Autodesk Fusion 360 part; units mm, degrees
note: some values were not read from the file. Set by a fixed rule: which sketch regions a step uses.
(part 15 of 59)
  spline S83 degree 5 poles (-2.755, -18.3773) (-2.7539, -18.3749) (-2.7515, -18.37) (-2.748, -18.3627) (-2.7434, -18.353) (-2.7376, -18.3408) (-2.7319, -18.3287) (-2.7262, -18.3165) (-2.7205, -18.3044) (-2.7149, -18.2924) (-2.7092, -18.2803) (-2.7036, -18.2683) (-2.6981, -18.2563) (-2.6925, -18.2443) (-2.687, -18.2323) (-2.6815, -18.2204) (-2.6761, -18.2085) (-2.6707, -18.1966) (-2.6653, -18.1847) (-2.6599, -18.1728) (-2.6545, -18.161) (-2.6492, -18.1492) (-2.6439, -18.1374) (-2.6387, -18.1256) (-2.6335, -18.1139) (-2.6283, -18.1022) (-2.6231, -18.0905) (-2.6179, -18.0788) (-2.6128, -18.0672) (-2.6077, -18.0555) (-2.6027, -18.0439) (-2.5977, -18.0324) (-2.5927, -18.0208) (-2.5877, -18.0093) (-2.5827, -17.9978) (-2.5778, -17.9863) (-2.5729, -17.9749) (-2.5681, -17.9634) (-2.5632, -17.952) (-2.5584, -17.9407) (-2.5537, -17.9293) (-2.5489, -17.918) (-2.5442, -17.9067) (-2.5395, -17.8954) (-2.5348, -17.8841) (-2.5302, -17.8729) (-2.5256, -17.8617) (-2.521, -17.8506) (-2.5165, -17.8394) (-2.5119, -17.8283) (-2.5074, -17.8172) (-2.503, -17.8061) (-2.4985, -17.7951) (-2.4941, -17.7841) (-2.4897, -17.7731) (-2.4854, -17.7621) (-2.481, -17.7512) (-2.4767, -17.7403) (-2.4725, -17.7294) (-2.4682, -17.7186) (-2.464, -17.7078) (-2.4598, -17.697) (-2.4557, -17.6862) (-2.4515, -17.6755) (-2.4474, -17.6648) (-2.4433, -17.6541) (-2.4393, -17.6435) (-2.4353, -17.6329) (-2.4313, -17.6223) (-2.4273, -17.6118) (-2.4234, -17.6012) (-2.4194, -17.5907) (-2.4156, -17.5803) (-2.4117, -17.5699) (-2.4079, -17.5595) (-2.4041, -17.5491) (-2.4003, -17.5388) (-2.3965, -17.5284) (-2.3928, -17.5182) (-2.3891, -17.5079) (-2.3855, -17.4977) (-2.3818, -17.4875) (-2.3782, -17.4774) (-2.3746, -17.4673) (-2.3711, -17.4572) (-2.3675, -17.4471) (-2.364, -17.4371) (-2.3606, -17.4271) (-2.3571, -17.4172) (-2.3537, -17.4073) (-2.3503, -17.3974) (-2.3469, -17.3875) (-2.3436, -17.3777) (-2.3403, -17.368) (-2.337, -17.3582) (-2.3337, -17.3485) (-2.3305, -17.3388) (-2.3273, -17.3292) (-2.3241, -17.3196) (-2.321, -17.31) (-2.3178, -17.3005) (-2.3147, -17.291) (-2.3117, -17.2815) (-2.3086, -17.2721) (-2.3056, -17.2627) (-2.3026, -17.2534) (-2.2996, -17.2441) (-2.2967, -17.2348) (-2.2938, -17.2255) (-2.2909, -17.2163) (-2.288, -17.2072) (-2.2852, -17.1981) (-2.2824, -17.189) (-2.2796, -17.1799) (-2.2769, -17.1709) (-2.2741, -17.1619) (-2.2714, -17.153) (-2.2688, -17.1441) (-2.2661, -17.1353) (-2.2635, -17.1265) (-2.2609, -17.1177) (-2.2583, -17.109) (-2.2558, -17.1003) (-2.2533, -17.0917) (-2.2508, -17.083) (-2.2483, -17.0745) (-2.2458, -17.066) (-2.2434, -17.0575) (-2.241, -17.0491) (-2.2387, -17.0407) (-2.2363, -17.0323) (-2.234, -17.024) (-2.2317, -17.0158) (-2.2295, -17.0075) (-2.2272, -16.9994) (-2.225, -16.9912) (-2.2228, -16.9832) (-2.2207, -16.9751) (-2.2185, -16.9671) (-2.2164, -16.9592) (-2.2143, -16.9513) (-2.2123, -16.9434) (-2.2102, -16.9356) (-2.2082, -16.9279) (-2.2062, -16.9202) (-2.2043, -16.9125) (-2.2023, -16.9049) (-2.2004, -16.8973) (-2.1985, -16.8898) (-2.1967, -16.8823) (-2.1948, -16.8749) (-2.193, -16.8675) (-2.1912, -16.8602) (-2.1895, -16.8529) (-2.1877, -16.8457) (-2.186, -16.8386) (-2.1843, -16.8314) (-2.1827, -16.8244) (-2.181, -16.8174) (-2.1794, -16.8104) (-2.1778, -16.8035) (-2.1762, -16.7967) (-2.1747, -16.7899) (-2.1731, -16.7831) (-2.1716, -16.7764) (-2.1702, -16.7698) (-2.1687, -16.7632) (-2.1673, -16.7567) (-2.1659, -16.7502) (-2.1645, -16.7438) (-2.1631, -16.7374) (-2.1618, -16.7311) (-2.1605, -16.7249) (-2.1592, -16.7187) (-2.1579, -16.7126) (-2.1567, -16.7065) (-2.1554, -16.7005) (-2.1542, -16.6946) (-2.153, -16.6887) (-2.1519, -16.6829) (-2.1507, -16.6771) (-2.1496, -16.6714) (-2.1485, -16.6658) (-2.1475, -16.6602) (-2.1464, -16.6547) (-2.1454, -16.6493) (-2.1444, -16.6439) (-2.1434, -16.6386) (-2.1424, -16.6334) (-2.1415, -16.6282) (-2.1406, -16.6231) (-2.1397, -16.618) (-2.1388, -16.6131) (-2.138, -16.6081) (-2.1371, -16.6033) (-2.1363, -16.5985) (-2.1355, -16.5938) (-2.1347, -16.5892) (-2.134, -16.5847) (-2.1332, -16.5802) (-2.1325, -16.5758) (-2.1318, -16.5714) (-2.1312, -16.5672) (-2.1305, -16.563) (-2.1299, -16.5589) (-2.1292, -16.5549) (-2.1286, -16.5509) (-2.1281, -16.547) (-2.1275, -16.5432) (-2.127, -16.5395) (-2.1264, -16.5359) (-2.1259, -16.5323) (-2.1254, -16.5289) (-2.125, -16.5255) (-2.1245, -16.5222) (-2.1241, -16.5189) (-2.1237, -16.5158) (-2.1233, -16.5128) (-2.1229, -16.5098) (-2.1225, -16.5069) (-2.1222, -16.5041) (-2.1219, -16.5015) (-2.1215, -16.4989) (-2.1212, -16.4963) (-2.121, -16.4939) (-2.1207, -16.4916) (-2.1204, -16.4894) (-2.1202, -16.4873) (-2.12, -16.4852) (-2.1198, -16.4833) (-2.1196, -16.4815) (-2.1194, -16.4798) (-2.1192, -16.4781) (-2.1191, -16.4766) (-2.1189, -16.4752) (-2.1188, -16.4739) (-2.1187, -16.4727) (-2.1186, -16.4716) (-2.1185, -16.4706) (-2.1184, -16.4698) (-2.1184, -16.469) (-2.1183, -16.4685) (-2.1183, -16.4682) (-2.1183, -16.468) (-2.1183, -16.4679) knots -1 -1 -1 -1 -1 -1 -0.99583333 -0.99166667 -0.9875 -0.98333333 -0.97916667 -0.975 -0.97083333 -0.96666667 -0.9625 -0.95833333 -0.95416667 -0.95 -0.94583333 -0.94166667 -0.9375 -0.93333333 -0.92916667 -0.925 -0.92083333 -0.91666667 -0.9125 -0.90833333 -0.90416667 -0.9 -0.89583333 -0.89166667 -0.8875 -0.88333333 -0.87916667 -0.875 -0.87083333 -0.86666667 -0.8625 -0.85833333 -0.85416667 -0.85 -0.84583333 -0.84166667 -0.8375 -0.83333333 -0.82916667 -0.825 -0.82083333 -0.81666667 -0.8125 -0.80833333 -0.80416667 -0.8 -0.79583333 -0.79166667 -0.7875 -0.78333333 -0.77916667 -0.775 -0.77083333 -0.76666667 -0.7625 -0.75833333 -0.75416667 -0.75 -0.74583333 -0.74166667 -0.7375 -0.73333333 -0.72916667 -0.725 -0.72083333 -0.71666667 -0.7125 -0.70833333 -0.70416667 -0.7 -0.69583333 -0.69166667 -0.6875 -0.68333333 -0.67916667 -0.675 -0.67083333 -0.66666667 -0.6625 -0.65833333 -0.65416667 -0.65 -0.64583333 -0.64166667 -0.6375 -0.63333333 -0.62916667 -0.625 -0.62083333 -0.61666667 -0.6125 -0.60833333 -0.60416667 -0.6 -0.59583333 -0.59166667 -0.5875 -0.58333333 -0.57916667 -0.575 -0.57083333 -0.56666667 -0.5625 -0.55833333 -0.55416667 -0.55 -0.54583333 -0.54166667 -0.5375 -0.53333333 -0.52916667 -0.525 -0.52083333 -0.51666667 -0.5125 -0.50833333 -0.50416667 -0.5 -0.49583333 -0.49166667 -0.4875 -0.48333333 -0.47916667 -0.475 -0.47083333 -0.46666667 -0.4625 -0.45833333 -0.45416667 -0.45 -0.44583333 -0.44166667 -0.4375 -0.43333333 -0.42916667 -0.425 -0.42083333 -0.41666667 -0.4125 -0.40833333 -0.40416667 -0.4 -0.39583333 -0.39166667 -0.3875 -0.38333333 -0.37916667 -0.375 -0.37083333 -0.36666667 -0.3625 -0.35833333 -0.35416667 -0.35 -0.34583333 -0.34166667 -0.3375 -0.33333333 -0.32916667 -0.325 -0.32083333 -0.31666667 -0.3125 -0.30833333 -0.30416667 -0.3 -0.29583333 -0.29166667 -0.2875 -0.28333333 -0.27916667 -0.275 -0.27083333 -0.26666667 -0.2625 -0.25833333 -0.25416667 -0.25 -0.24583333 -0.24166667 -0.2375 -0.23333333 -0.22916667 -0.225 -0.22083333 -0.21666667 -0.2125 -0.20833333 -0.20416667 -0.2 -0.19583333 -0.19166667 -0.1875 -0.18333333 -0.17916667 -0.175 -0.17083333 -0.16666667 -0.1625 -0.15833333 -0.15416667 -0.15 -0.14583333 -0.14166667 -0.1375 -0.13333333 -0.12916667 -0.125 -0.12083333 -0.11666667 -0.1125 -0.10833333 -0.10416667 -0.1 -0.09583333 -0.09166667 -0.0875 -0.08333333 -0.07916667 -0.075 -0.07083333 -0.06666667 -0.0625 -0.05833333 -0.05416667 -0.05 -0.04583333 -0.04166667 -0.0375 -0.03333333 -0.02916667 -0.025 -0.02083333 -0.01666667 -0.0125 -0.00833333 -0.00416667 0 0 0 0 0 0
  spline S84 degree 5 poles (26.1461, -0.1495) (26.1462, -0.1495) (26.1464, -0.1496) (26.1467, -0.1497) (26.1471, -0.15) (26.1478, -0.1503) (26.1486, -0.1506) (26.1495, -0.151) (26.1504, -0.1515) (26.1515, -0.152) (26.1527, -0.1526) (26.154, -0.1531) (26.1554, -0.1538) (26.1569, -0.1544) (26.1585, -0.1551) (26.1602, -0.1559) (26.1619, -0.1567) (26.1638, -0.1575) (26.1658, -0.1583) (26.1678, -0.1592) (26.17, -0.1602) (26.1722, -0.1611) (26.1745, -0.1621) (26.1769, -0.1631) (26.1794, -0.1642) (26.182, -0.1653) (26.1847, -0.1664) (26.1874, -0.1676) (26.1903, -0.1687) (26.1932, -0.1699) (26.1962, -0.1712) (26.1993, -0.1724) (26.2024, -0.1737) (26.2057, -0.175) (26.209, -0.1764) (26.2124, -0.1778) (26.2159, -0.1791) (26.2195, -0.1806) (26.2231, -0.182) (26.2269, -0.1834) (26.2307, -0.1849) (26.2345, -0.1864) (26.2385, -0.188) (26.2425, -0.1895) (26.2466, -0.1911) (26.2508, -0.1927) (26.255, -0.1943) (26.2594, -0.1959) (26.2638, -0.1975) (26.2682, -0.1992) (26.2728, -0.2009) (26.2774, -0.2026) (26.282, -0.2043) (26.2868, -0.206) (26.2916, -0.2077) (26.2965, -0.2095) (26.3015, -0.2113) (26.3065, -0.2131) (26.3116, -0.2149) (26.3167, -0.2167) (26.322, -0.2185) (26.3273, -0.2204) (26.3326, -0.2222) (26.338, -0.2241) (26.3435, -0.226) (26.3491, -0.2279) (26.3547, -0.2298) (26.3604, -0.2317) (26.3661, -0.2336) (26.3719, -0.2356) (26.3778, -0.2375) (26.3837, -0.2395) (26.3897, -0.2414) (26.3958, -0.2434) (26.4019, -0.2454) (26.4081, -0.2474) (26.4144, -0.2494) (26.4207, -0.2514) (26.427, -0.2534) (26.4335, -0.2555) (26.4399, -0.2575) (26.4465, -0.2596) (26.4531, -0.2616) (26.4598, -0.2637) (26.4665, -0.2657) (26.4733, -0.2678) (26.4801, -0.2699) (26.487, -0.272) (26.4939, -0.274) (26.5009, -0.2761) (26.508, -0.2782) (26.5151, -0.2803) (26.5223, -0.2824) (26.5296, -0.2845) (26.5368, -0.2867) (26.5442, -0.2888) (26.5516, -0.2909) (26.559, -0.293) (26.5665, -0.2952) (26.5741, -0.2973) (26.5817, -0.2994) (26.5894, -0.3016) (26.5971, -0.3037) (26.6049, -0.3058) (26.6127, -0.308) (26.6206, -0.3101) (26.6286, -0.3123) (26.6365, -0.3144) (26.6446, -0.3166) (26.6527, -0.3187) (26.6608, -0.3208) (26.669, -0.323) (26.6773, -0.3251) (26.6856, -0.3273) (26.6939, -0.3294) (26.7023, -0.3316) (26.7108, -0.3337) (26.7193, -0.3359) (26.7278, -0.338) (26.7364, -0.3402) (26.7451, -0.3423) (26.7537, -0.3445) (26.7625, -0.3466) (26.7713, -0.3487) (26.7801, -0.3509) (26.789, -0.353) (26.798, -0.3551) (26.8069, -0.3573) (26.816, -0.3594) (26.8251, -0.3615) (26.8342, -0.3636) (26.8434, -0.3658) (26.8526, -0.3679) (26.8619, -0.37) (26.8712, -0.3721) (26.8806, -0.3742) (26.89, -0.3763) (26.8994, -0.3784) (26.9089, -0.3805) (26.9185, -0.3826) (26.9281, -0.3847) (26.9377, -0.3867) (26.9474, -0.3888) (26.9571, -0.3909) (26.9669, -0.3929) (26.9767, -0.395) (26.9866, -0.3971) (26.9965, -0.3991) (27.0064, -0.4011) (27.0164, -0.4032) (27.0265, -0.4052) (27.0365, -0.4072) (27.0467, -0.4093) (27.0568, -0.4113) (27.0671, -0.4133) (27.0773, -0.4153) (27.0876, -0.4173) (27.0979, -0.4193) (27.1083, -0.4213) (27.1188, -0.4232) (27.1292, -0.4252) (27.1397, -0.4272) (27.1503, -0.4291) (27.1609, -0.4311) (27.1715, -0.433) (27.1822, -0.4349) (27.1929, -0.4368) (27.2037, -0.4388) (27.2145, -0.4407) (27.2253, -0.4426) (27.2362, -0.4445) (27.2471, -0.4463) (27.2581, -0.4482) (27.2691, -0.4501) (27.2801, -0.4519) (27.2912, -0.4538) (27.3023, -0.4556) (27.3135, -0.4574) (27.3247, -0.4593) (27.3359, -0.4611) (27.3472, -0.4629) (27.3585, -0.4647) (27.3699, -0.4665) (27.3813, -0.4682) (27.3927, -0.47) (27.4042, -0.4718) (27.4157, -0.4735) (27.4273, -0.4752) (27.4388, -0.477) (27.4505, -0.4787) (27.4621, -0.4804) (27.4738, -0.4821) (27.4856, -0.4838) (27.4974, -0.4854) (27.5092, -0.4871) (27.521, -0.4887) (27.5329, -0.4904) (27.5449, -0.492) (27.5568, -0.4936) (27.5688, -0.4952) (27.5809, -0.4968) (27.5929, -0.4984) (27.605, -0.5) (27.6172, -0.5016) (27.6294, -0.5031) (27.6416, -0.5047) (27.6539, -0.5062) (27.6661, -0.5077) (27.6785, -0.5092) (27.6908, -0.5107) (27.7032, -0.5122) (27.7157, -0.5136) (27.7281, -0.5151) (27.7406, -0.5165) (27.7532, -0.518) (27.7658, -0.5194) (27.7784, -0.5208) (27.791, -0.5222) (27.8037, -0.5236) (27.8164, -0.5249) (27.8291, -0.5263) (27.8419, -0.5276) (27.8547, -0.529) (27.8676, -0.5303) (27.8805, -0.5316) (27.8934, -0.5329) (27.9063, -0.5342) (27.9193, -0.5354) (27.9323, -0.5367) (27.9454, -0.5379) (27.9585, -0.5391) (27.9716, -0.5404) (27.9848, -0.5415) (27.9979, -0.5427) (28.0112, -0.5439) (28.0244, -0.5451) (28.0377, -0.5462) (28.051, -0.5473) (28.0644, -0.5484) (28.0777, -0.5495) (28.0911, -0.5506) (28.1019, -0.5515) (28.11, -0.5521) (28.1154, -0.5525) (28.1181, -0.5527) knots 0 0 0 0 0 0 0.00416667 0.00833333 0.0125 0.01666667 0.02083333 0.025 0.02916667 0.03333333 0.0375 0.04166667 0.04583333 0.05 0.05416667 0.05833333 0.0625 0.06666667 0.07083333 0.075 0.07916667 0.08333333 0.0875 0.09166667 0.09583333 0.1 0.10416667 0.10833333 0.1125 0.11666667 0.12083333 0.125 0.12916667 0.13333333 0.1375 0.14166667 0.14583333 0.15 0.15416667 0.15833333 0.1625 0.16666667 0.17083333 0.175 0.17916667 0.18333333 0.1875 0.19166667 0.19583333 0.2 0.20416667 0.20833333 0.2125 0.21666667 0.22083333 0.225 0.22916667 0.23333333 0.2375 0.24166667 0.24583333 0.25 0.25416667 0.25833333 0.2625 0.26666667 0.27083333 0.275 0.27916667 0.28333333 0.2875 0.29166667 0.29583333 0.3 0.30416667 0.30833333 0.3125 0.31666667 0.32083333 0.325 0.32916667 0.33333333 0.3375 0.34166667 0.34583333 0.35 0.35416667 0.35833333 0.3625 0.36666667 0.37083333 0.375 0.37916667 0.38333333 0.3875 0.39166667 0.39583333 0.4 0.40416667 0.40833333 0.4125 0.41666667 0.42083333 0.425 0.42916667 0.43333333 0.4375 0.44166667 0.44583333 0.45 0.45416667 0.45833333 0.4625 0.46666667 0.47083333 0.475 0.47916667 0.48333333 0.4875 0.49166667 0.49583333 0.5 0.50416667 0.50833333 0.5125 0.51666667 0.52083333 0.525 0.52916667 0.53333333 0.5375 0.54166667 0.54583333 0.55 0.55416667 0.55833333 0.5625 0.56666667 0.57083333 0.575 0.57916667 0.58333333 0.5875 0.59166667 0.59583333 0.6 0.60416667 0.60833333 0.6125 0.61666667 0.62083333 0.625 0.62916667 0.63333333 0.6375 0.64166667 0.64583333 0.65 0.65416667 0.65833333 0.6625 0.66666667 0.67083333 0.675 0.67916667 0.68333333 0.6875 0.69166667 0.69583333 0.7 0.70416667 0.70833333 0.7125 0.71666667 0.72083333 0.725 0.72916667 0.73333333 0.7375 0.74166667 0.74583333 0.75 0.75416667 0.75833333 0.7625 0.76666667 0.77083333 0.775 0.77916667 0.78333333 0.7875 0.79166667 0.79583333 0.8 0.80416667 0.80833333 0.8125 0.81666667 0.82083333 0.825 0.82916667 0.83333333 0.8375 0.84166667 0.84583333 0.85 0.85416667 0.85833333 0.8625 0.86666667 0.87083333 0.875 0.87916667 0.88333333 0.8875 0.89166667 0.89583333 0.9 0.90416667 0.90833333 0.9125 0.91666667 0.92083333 0.925 0.92916667 0.93333333 0.9375 0.94166667 0.94583333 0.95 0.95416667 0.95833333 0.9625 0.96666667 0.97083333 0.975 0.97916667 0.98333333 0.9875 0.99166667 0.99583333 1 1 1 1 1 1
  arc A88 (18.6136, 37.2898) -> (17.8246, 37.863) centre (0, 12.5) ccw
  spline S85 degree 5 poles (5.9675, 42.9202) (5.9661, 42.9179) (5.9633, 42.9133) (5.959, 42.9064) (5.9534, 42.8972) (5.9464, 42.8857) (5.9394, 42.8742) (5.9325, 42.8628) (5.9255, 42.8513) (5.9187, 42.8399) (5.9118, 42.8285) (5.905, 42.8171) (5.8982, 42.8058) (5.8914, 42.7944) (5.8847, 42.7831) (5.878, 42.7718) (5.8713, 42.7605) (5.8647, 42.7492) (5.8581, 42.738) (5.8515, 42.7268) (5.8449, 42.7156) (5.8384, 42.7044) (5.8319, 42.6932) (5.8255, 42.6821) (5.8191, 42.6709) (5.8127, 42.6598) (5.8063, 42.6487) (5.8, 42.6377) (5.7937, 42.6266) (5.7874, 42.6156) (5.7811, 42.6046) (5.7749, 42.5936) (5.7688, 42.5826) (5.7626, 42.5717) (5.7565, 42.5608) (5.7504, 42.5499) (5.7443, 42.539) (5.7383, 42.5281) (5.7323, 42.5173) (5.7263, 42.5065) (5.7204, 42.4957) (5.7145, 42.4849) (5.7086, 42.4742) (5.7028, 42.4634) (5.697, 42.4527) (5.6912, 42.4421) (5.6854, 42.4314) (5.6797, 42.4208) (5.674, 42.4102) (5.6683, 42.3996) (5.6627, 42.389) (5.6571, 42.3785) (5.6515, 42.368) (5.646, 42.3575) (5.6405, 42.347) (5.635, 42.3366) (5.6296, 42.3262) (5.6242, 42.3158) (5.6188, 42.3054) (5.6134, 42.2951) (5.6081, 42.2847) (5.6028, 42.2745) (5.5975, 42.2642) (5.5923, 42.254) (5.5871, 42.2437) (5.5819, 42.2336) (5.5768, 42.2234) (5.5717, 42.2133) (5.5666, 42.2032) (5.5615, 42.1931) (5.5565, 42.183) (5.5515, 42.173) (5.5466, 42.163) (5.5416, 42.153) (5.5367, 42.1431) (5.5319, 42.1332) (5.527, 42.1233) (5.5222, 42.1134) (5.5175, 42.1036) (5.5127, 42.0938) (5.508, 42.084) (5.5033, 42.0743) (5.4987, 42.0646) (5.494, 42.0549) (5.4895, 42.0452) (5.4849, 42.0356) (5.4804, 42.026) (5.4759, 42.0165) (5.4714, 42.0069) (5.467, 41.9974) (5.4625, 41.9879) (5.4582, 41.9785) (5.4538, 41.9691) (5.4495, 41.9597) (5.4452, 41.9504) (5.441, 41.941) (5.4367, 41.9318) (5.4325, 41.9225) (5.4284, 41.9133) (5.4242, 41.9041) (5.4201, 41.895) (5.4161, 41.8858) (5.412, 41.8767) (5.408, 41.8677) (5.404, 41.8587) (5.4001, 41.8497) (5.3961, 41.8407) (5.3922, 41.8318) (5.3884, 41.8229) (5.3846, 41.8141) (5.3807, 41.8053) (5.377, 41.7965) (5.3732, 41.7878) (5.3695, 41.779) (5.3658, 41.7704) (5.3622, 41.7617) (5.3586, 41.7531) (5.355, 41.7446) (5.3514, 41.7361) (5.3479, 41.7276) (5.3444, 41.7191) (5.3409, 41.7107) (5.3375, 41.7023) (5.3341, 41.694) (5.3307, 41.6857) (5.3273, 41.6775) (5.324, 41.6692) (5.3207, 41.6611) (5.3175, 41.6529) (5.3143, 41.6448) (5.3111, 41.6368) (5.3079, 41.6288) (5.3047, 41.6208) (5.3016, 41.6129) (5.2986, 41.605) (5.2955, 41.5971) (5.2925, 41.5893) (5.2895, 41.5815) (5.2865, 41.5738) (5.2836, 41.5661) (5.2807, 41.5585) (5.2778, 41.5509) (5.275, 41.5433) (5.2722, 41.5358) (5.2694, 41.5284) (5.2666, 41.521) (5.2639, 41.5136) (5.2612, 41.5063) (5.2586, 41.499) (5.2559, 41.4918) (5.2533, 41.4846) (5.2508, 41.4774) (5.2482, 41.4703) (5.2457, 41.4633) (5.2432, 41.4563) (5.2408, 41.4493) (5.2383, 41.4424) (5.2359, 41.4356) (5.2336, 41.4288) (5.2312, 41.422) (5.2289, 41.4153) (5.2266, 41.4087) (5.2244, 41.4021) (5.2222, 41.3955) (5.22, 41.389) (5.2178, 41.3826) (5.2157, 41.3762) (5.2136, 41.3699) (5.2115, 41.3636) (5.2094, 41.3573) (5.2074, 41.3512) (5.2054, 41.3451) (5.2035, 41.339) (5.2015, 41.333) (5.1996, 41.327) (5.1978, 41.3211) (5.1959, 41.3153) (5.1941, 41.3095) (5.1923, 41.3038) (5.1905, 41.2981) (5.1888, 41.2925) (5.1871, 41.2869) (5.1854, 41.2815) (5.1838, 41.276) (5.1822, 41.2707) (5.1806, 41.2654) (5.179, 41.2601) (5.1775, 41.2549) (5.176, 41.2498) (5.1745, 41.2448) (5.173, 41.2398) (5.1716, 41.2349) (5.1702, 41.23) (5.1689, 41.2252) (5.1675, 41.2205) (5.1662, 41.2158) (5.1649, 41.2112) (5.1637, 41.2067) (5.1625, 41.2023) (5.1613, 41.1979) (5.1601, 41.1936) (5.1589, 41.1893) (5.1578, 41.1852) (5.1567, 41.1811) (5.1557, 41.1771) (5.1546, 41.1731) (5.1536, 41.1693) (5.1527, 41.1655) (5.1517, 41.1617) (5.1508, 41.1581) (5.1499, 41.1545) (5.149, 41.1511) (5.1481, 41.1477) (5.1473, 41.1443) (5.1465, 41.1411) (5.1458, 41.1379) (5.145, 41.1349) (5.1443, 41.1319) (5.1436, 41.129) (5.143, 41.1262) (5.1423, 41.1234) (5.1417, 41.1208) (5.1411, 41.1182) (5.1406, 41.1158) (5.14, 41.1134) (5.1395, 41.1111) (5.139, 41.1089) (5.1386, 41.1069) (5.1381, 41.1049) (5.1377, 41.103) (5.1374, 41.1012) (5.137, 41.0995) (5.1367, 41.0979) (5.1363, 41.0964) (5.1361, 41.095) (5.1358, 41.0937) (5.1356, 41.0925) (5.1354, 41.0915) (5.1352, 41.0905) (5.135, 41.0896) (5.1349, 41.0889) (5.1348, 41.0884) (5.1347, 41.0881) (5.1347, 41.0879) (5.1346, 41.0878) knots -1 -1 -1 -1 -1 -1 -0.99583333 -0.99166667 -0.9875 -0.98333333 -0.97916667 -0.975 -0.97083333 -0.96666667 -0.9625 -0.95833333 -0.95416667 -0.95 -0.94583333 -0.94166667 -0.9375 -0.93333333 -0.92916667 -0.925 -0.92083333 -0.91666667 -0.9125 -0.90833333 -0.90416667 -0.9 -0.89583333 -0.89166667 -0.8875 -0.88333333 -0.87916667 -0.875 -0.87083333 -0.86666667 -0.8625 -0.85833333 -0.85416667 -0.85 -0.84583333 -0.84166667 -0.8375 -0.83333333 -0.82916667 -0.825 -0.82083333 -0.81666667 -0.8125 -0.80833333 -0.80416667 -0.8 -0.79583333 -0.79166667 -0.7875 -0.78333333 -0.77916667 -0.775 -0.77083333 -0.76666667 -0.7625 -0.75833333 -0.75416667 -0.75 -0.74583333 -0.74166667 -0.7375 -0.73333333 -0.72916667 -0.725 -0.72083333 -0.71666667 -0.7125 -0.70833333 -0.70416667 -0.7 -0.69583333 -0.69166667 -0.6875 -0.68333333 -0.67916667 -0.675 -0.67083333 -0.66666667 -0.6625 -0.65833333 -0.65416667 -0.65 -0.64583333 -0.64166667 -0.6375 -0.63333333 -0.62916667 -0.625 -0.62083333 -0.61666667 -0.6125 -0.60833333 -0.60416667 -0.6 -0.59583333 -0.59166667 -0.5875 -0.58333333 -0.57916667 -0.575 -0.57083333 -0.56666667 -0.5625 -0.55833333 -0.55416667 -0.55 -0.54583333 -0.54166667 -0.5375 -0.53333333 -0.52916667 -0.525 -0.52083333 -0.51666667 -0.5125 -0.50833333 -0.50416667 -0.5 -0.49583333 -0.49166667 -0.4875 -0.48333333 -0.47916667 -0.475 -0.47083333 -0.46666667 -0.4625 -0.45833333 -0.45416667 -0.45 -0.44583333 -0.44166667 -0.4375 -0.43333333 -0.42916667 -0.425 -0.42083333 -0.41666667 -0.4125 -0.40833333 -0.40416667 -0.4 -0.39583333 -0.39166667 -0.3875 -0.38333333 -0.37916667 -0.375 -0.37083333 -0.36666667 -0.3625 -0.35833333 -0.35416667 -0.35 -0.34583333 -0.34166667 -0.3375 -0.33333333 -0.32916667 -0.325 -0.32083333 -0.31666667 -0.3125 -0.30833333 -0.30416667 -0.3 -0.29583333 -0.29166667 -0.2875 -0.28333333 -0.27916667 -0.275 -0.27083333 -0.26666667 -0.2625 -0.25833333 -0.25416667 -0.25 -0.24583333 -0.24166667 -0.2375 -0.23333333 -0.22916667 -0.225 -0.22083333 -0.21666667 -0.2125 -0.20833333 -0.20416667 -0.2 -0.19583333 -0.19166667 -0.1875 -0.18333333 -0.17916667 -0.175 -0.17083333 -0.16666667 -0.1625 -0.15833333 -0.15416667 -0.15 -0.14583333 -0.14166667 -0.1375 -0.13333333 -0.12916667 -0.125 -0.12083333 -0.11666667 -0.1125 -0.10833333 -0.10416667 -0.1 -0.09583333 -0.09166667 -0.0875 -0.08333333 -0.07916667 -0.075 -0.07083333 -0.06666667 -0.0625 -0.05833333 -0.05416667 -0.05 -0.04583333 -0.04166667 -0.0375 -0.03333333 -0.02916667 -0.025 -0.02083333 -0.01666667 -0.0125 -0.00833333 -0.00416667 0 0 0 0 0 0
  spline S86 degree 5 poles (28.7753, 8.5492) (28.7754, 8.5492) (28.7756, 8.5492) (28.7759, 8.5491) (28.7764, 8.5491) (28.7772, 8.549) (28.778, 8.5489) (28.779, 8.5488) (28.7801, 8.5486) (28.7813, 8.5485) (28.7826, 8.5483) (28.784, 8.5482) (28.7855, 8.548) (28.7871, 8.5478) (28.7889, 8.5477) (28.7907, 8.5475) (28.7926, 8.5473) (28.7946, 8.5471) (28.7968, 8.5469) (28.799, 8.5466) (28.8013, 8.5464) (28.8037, 8.5462) (28.8063, 8.546) (28.8089, 8.5457) (28.8116, 8.5455) (28.8144, 8.5453) (28.8172, 8.545) (28.8202, 8.5448) (28.8233, 8.5445) (28.8264, 8.5443) (28.8297, 8.5441) (28.833, 8.5438) (28.8364, 8.5436) (28.8399, 8.5433) (28.8435, 8.5431) (28.8472, 8.5428) (28.8509, 8.5426) (28.8547, 8.5423) (28.8586, 8.5421) (28.8626, 8.5419) (28.8667, 8.5416) (28.8709, 8.5414) (28.8751, 8.5412) (28.8794, 8.541) (28.8838, 8.5407) (28.8882, 8.5405) (28.8928, 8.5403) (28.8974, 8.5401) (28.9021, 8.5399) (28.9068, 8.5397) (28.9117, 8.5395) (28.9166, 8.5393) (28.9215, 8.5391) (28.9266, 8.539) (28.9317, 8.5388) (28.9369, 8.5386) (28.9422, 8.5385) (28.9475, 8.5383) (28.9529, 8.5382) (28.9584, 8.538) (28.9639, 8.5379) (28.9695, 8.5378) (28.9752, 8.5377) (28.9809, 8.5376) (28.9867, 8.5375) (28.9926, 8.5374) (28.9985, 8.5373) (29.0045, 8.5373) (29.0106, 8.5372) (29.0167, 8.5371) (29.0229, 8.5371) (29.0291, 8.5371) (29.0355, 8.5371) (29.0418, 8.537) (29.0483, 8.537) (29.0548, 8.5371) (29.0613, 8.5371) (29.068, 8.5371) (29.0746, 8.5372) (29.0814, 8.5372) (29.0882, 8.5373) (29.095, 8.5374) (29.1019, 8.5374) (29.1089, 8.5375) (29.1159, 8.5377) (29.123, 8.5378) (29.1302, 8.5379) (29.1374, 8.5381) (29.1446, 8.5382) (29.1519, 8.5384) (29.1593, 8.5386) (29.1667, 8.5388) (29.1742, 8.539) (29.1817, 8.5393) (29.1893, 8.5395) (29.197, 8.5397) (29.2047, 8.54) (29.2124, 8.5403) (29.2202, 8.5406) (29.2281, 8.5409) (29.236, 8.5412) (29.2439, 8.5416) (29.2519, 8.5419) (29.26, 8.5423) (29.2681, 8.5427) (29.2763, 8.5431) (29.2845, 8.5435) (29.2927, 8.5439) (29.301, 8.5444) (29.3094, 8.5448) (29.3178, 8.5453) (29.3263, 8.5458) (29.3348, 8.5463) (29.3433, 8.5468) (29.3519, 8.5474) (29.3606, 8.5479) (29.3693, 8.5485) (29.378, 8.5491) (29.3868, 8.5497) (29.3957, 8.5503) (29.4045, 8.5509) (29.4135, 8.5516) (29.4225, 8.5522) (29.4315, 8.5529) (29.4406, 8.5536) (29.4497, 8.5543) (29.4588, 8.5551) (29.468, 8.5558) (29.4773, 8.5566) (29.4866, 8.5574) (29.4959, 8.5582) (29.5053, 8.559) (29.5147, 8.5598) (29.5242, 8.5607) (29.5337, 8.5616) (29.5433, 8.5625) (29.5529, 8.5634) (29.5625, 8.5643) (29.5722, 8.5652) (29.5819, 8.5662) (29.5917, 8.5672) (29.6015, 8.5682) (29.6113, 8.5692) (29.6212, 8.5703) (29.6312, 8.5713) (29.6411, 8.5724) (29.6512, 8.5735) (29.6612, 8.5746) (29.6713, 8.5757) (29.6814, 8.5769) (29.6916, 8.578) (29.7018, 8.5792) (29.7121, 8.5804) (29.7224, 8.5817) (29.7327, 8.5829) (29.7431, 8.5842) (29.7535, 8.5855) (29.764, 8.5868) (29.7744, 8.5881) (29.785, 8.5894) (29.7955, 8.5908) (29.8061, 8.5922) (29.8168, 8.5936) (29.8274, 8.595) (29.8382, 8.5965) (29.8489, 8.5979) (29.8597, 8.5994) (29.8705, 8.6009) (29.8814, 8.6024) (29.8923, 8.604) (29.9032, 8.6055) (29.9142, 8.6071) (29.9252, 8.6087) (29.9362, 8.6104) (29.9473, 8.612) (29.9584, 8.6137) (29.9696, 8.6154) (29.9807, 8.6171) (29.992, 8.6188) (30.0032, 8.6205) (30.0145, 8.6223) (30.0258, 8.6241) (30.0372, 8.6259) (30.0486, 8.6278) (30.06, 8.6296) (30.0714, 8.6315) (30.0829, 8.6334) (30.0944, 8.6353) (30.106, 8.6372) (30.1176, 8.6392) (30.1292, 8.6412) (30.1409, 8.6432) (30.1525, 8.6452) (30.1643, 8.6473) (30.176, 8.6493) (30.1878, 8.6514) (30.1996, 8.6536) (30.2115, 8.6557) (30.2233, 8.6578) (30.2353, 8.66) (30.2472, 8.6622) (30.2592, 8.6644) (30.2712, 8.6667) (30.2832, 8.669) (30.2953, 8.6712) (30.3074, 8.6736) (30.3195, 8.6759) (30.3317, 8.6783) (30.3439, 8.6806) (30.3561, 8.683) (30.3683, 8.6855) (30.3806, 8.6879) (30.3929, 8.6904) (30.4053, 8.6929) (30.4176, 8.6954) (30.43, 8.6979) (30.4424, 8.7005) (30.4549, 8.703) (30.4674, 8.7057) (30.4799, 8.7083) (30.4924, 8.7109) (30.505, 8.7136) (30.5176, 8.7163) (30.5302, 8.719) (30.5429, 8.7218) (30.5556, 8.7245) (30.5683, 8.7273) (30.581, 8.7301) (30.5938, 8.733) (30.6066, 8.7358) (30.6194, 8.7387) (30.6323, 8.7416) (30.6451, 8.7445) (30.658, 8.7475) (30.671, 8.7504) (30.6839, 8.7534) (30.6969, 8.7565) (30.7099, 8.7595) (30.723, 8.7626) (30.736, 8.7657) (30.7491, 8.7688) (30.7596, 8.7713) (30.7675, 8.7732) (30.7728, 8.7744) (30.7754, 8.7751) knots 0 0 0 0 0 0 0.00416667 0.00833333 0.0125 0.01666667 0.02083333 0.025 0.02916667 0.03333333 0.0375 0.04166667 0.04583333 0.05 0.05416667 0.05833333 0.0625 0.06666667 0.07083333 0.075 0.07916667 0.08333333 0.0875 0.09166667 0.09583333 0.1 0.10416667 0.10833333 0.1125 0.11666667 0.12083333 0.125 0.12916667 0.13333333 0.1375 0.14166667 0.14583333 0.15 0.15416667 0.15833333 0.1625 0.16666667 0.17083333 0.175 0.17916667 0.18333333 0.1875 0.19166667 0.19583333 0.2 0.20416667 0.20833333 0.2125 0.21666667 0.22083333 0.225 0.22916667 0.23333333 0.2375 0.24166667 0.24583333 0.25 0.25416667 0.25833333 0.2625 0.26666667 0.27083333 0.275 0.27916667 0.28333333 0.2875 0.29166667 0.29583333 0.3 0.30416667 0.30833333 0.3125 0.31666667 0.32083333 0.325 0.32916667 0.33333333 0.3375 0.34166667 0.34583333 0.35 0.35416667 0.35833333 0.3625 0.36666667 0.37083333 0.375 0.37916667 0.38333333 0.3875 0.39166667 0.39583333 0.4 0.40416667 0.40833333 0.4125 0.41666667 0.42083333 0.425 0.42916667 0.43333333 0.4375 0.44166667 0.44583333 0.45 0.45416667 0.45833333 0.4625 0.46666667 0.47083333 0.475 0.47916667 0.48333333 0.4875 0.49166667 0.49583333 0.5 0.50416667 0.50833333 0.5125 0.51666667 0.52083333 0.525 0.52916667 0.53333333 0.5375 0.54166667 0.54583333 0.55 0.55416667 0.55833333 0.5625 0.56666667 0.57083333 0.575 0.57916667 0.58333333 0.5875 0.59166667 0.59583333 0.6 0.60416667 0.60833333 0.6125 0.61666667 0.62083333 0.625 0.62916667 0.63333333 0.6375 0.64166667 0.64583333 0.65 0.65416667 0.65833333 0.6625 0.66666667 0.67083333 0.675 0.67916667 0.68333333 0.6875 0.69166667 0.69583333 0.7 0.70416667 0.70833333 0.7125 0.71666667 0.72083333 0.725 0.72916667 0.73333333 0.7375 0.74166667 0.74583333 0.75 0.75416667 0.75833333 0.7625 0.76666667 0.77083333 0.775 0.77916667 0.78333333 0.7875 0.79166667 0.79583333 0.8 0.80416667 0.80833333 0.8125 0.81666667 0.82083333 0.825 0.82916667 0.83333333 0.8375 0.84166667 0.84583333 0.85 0.85416667 0.85833333 0.8625 0.86666667 0.87083333 0.875 0.87916667 0.88333333 0.8875 0.89166667 0.89583333 0.9 0.90416667 0.90833333 0.9125 0.91666667 0.92083333 0.925 0.92916667 0.93333333 0.9375 0.94166667 0.94583333 0.95 0.95416667 0.95833333 0.9625 0.96666667 0.97083333 0.975 0.97916667 0.98333333 0.9875 0.99166667 0.99583333 1 1 1 1 1 1
  spline S87 degree 5 poles (10.0421, -16.8284) (10.0422, -16.8257) (10.0423, -16.8203) (10.0425, -16.8122) (10.0428, -16.8014) (10.0431, -16.788) (10.0434, -16.7745) (10.0437, -16.7612) (10.044, -16.7478) (10.0442, -16.7345) (10.0445, -16.7212) (10.0447, -16.7079) (10.0449, -16.6947) (10.0451, -16.6815) (10.0453, -16.6683) (10.0454, -16.6551) (10.0455, -16.642) (10.0457, -16.629) (10.0458, -16.6159) (10.0458, -16.6029) (10.0459, -16.5899) (10.046, -16.577) (10.046, -16.5641) (10.046, -16.5512) (10.046, -16.5383) (10.046, -16.5255) (10.046, -16.5127) (10.0459, -16.5) (10.0458, -16.4872) (10.0458, -16.4745) (10.0457, -16.4619) (10.0456, -16.4493) (10.0454, -16.4367) (10.0453, -16.4241) (10.0451, -16.4116) (10.0449, -16.3991) (10.0448, -16.3867) (10.0445, -16.3743) (10.0443, -16.3619) (10.0441, -16.3495) (10.0438, -16.3372) (10.0436, -16.3249) (10.0433, -16.3127) (10.043, -16.3005) (10.0427, -16.2883) (10.0423, -16.2762) (10.042, -16.2641) (10.0416, -16.252) (10.0412, -16.24) (10.0409, -16.228) (10.0405, -16.216) (10.04, -16.2041) (10.0396, -16.1922) (10.0392, -16.1803) (10.0387, -16.1685) (10.0382, -16.1567) (10.0377, -16.145) (10.0372, -16.1333) (10.0367, -16.1216) (10.0362, -16.11) (10.0356, -16.0984) (10.0351, -16.0868) (10.0345, -16.0753) (10.0339, -16.0638) (10.0333, -16.0524) (10.0327, -16.041) (10.0321, -16.0296) (10.0314, -16.0183) (10.0308, -16.007) (10.0301, -15.9957) (10.0294, -15.9845) (10.0287, -15.9733) (10.028, -15.9622) (10.0273, -15.9511) (10.0266, -15.94) (10.0258, -15.929) (10.0251, -15.9181) (10.0243, -15.9071) (10.0235, -15.8962) (10.0227, -15.8854) (10.0219, -15.8745) (10.0211, -15.8638) (10.0203, -15.853) (10.0195, -15.8423) (10.0186, -15.8317) (10.0177, -15.821) (10.0169, -15.8105) (10.016, -15.7999) (10.0151, -15.7894) (10.0142, -15.779) (10.0133, -15.7686) (10.0123, -15.7582) (10.0114, -15.7479) (10.0104, -15.7376) (10.0095, -15.7274) (10.0085, -15.7172) (10.0075, -15.707) (10.0065, -15.6969) (10.0055, -15.6868) (10.0045, -15.6768) (10.0035, -15.6668) (10.0025, -15.6569) (10.0014, -15.647) (10.0004, -15.6372) (9.9993, -15.6274) (9.9983, -15.6176) (9.9972, -15.6079) (9.9961, -15.5982) (9.995, -15.5886) (9.9939, -15.579) (9.9928, -15.5695) (9.9916, -15.56) (9.9905, -15.5506) (9.9894, -15.5412) (9.9882, -15.5318) (9.9871, -15.5225) (9.9859, -15.5133) (9.9847, -15.504) (9.9836, -15.4949) (9.9824, -15.4858) (9.9812, -15.4767) (9.98, -15.4677) (9.9788, -15.4587) (9.9776, -15.4498) (9.9763, -15.4409) (9.9751, -15.4321) (9.9739, -15.4233) (9.9726, -15.4146) (9.9714, -15.4059) (9.9701, -15.3973) (9.9689, -15.3887) (9.9676, -15.3802) (9.9664, -15.3717) (9.9651, -15.3633) (9.9638, -15.3549) (9.9625, -15.3466) (9.9612, -15.3383) (9.9599, -15.3301) (9.9586, -15.3219) (9.9573, -15.3138) (9.956, -15.3057) (9.9547, -15.2977) (9.9534, -15.2898) (9.9521, -15.2819) (9.9508, -15.274) (9.9494, -15.2662) (9.9481, -15.2585) (9.9468, -15.2508) (9.9454, -15.2431) (9.9441, -15.2356) (9.9428, -15.228) (9.9414, -15.2206) (9.9401, -15.2132) (9.9387, -15.2058) (9.9374, -15.1985) (9.936, -15.1912) (9.9347, -15.1841) (9.9333, -15.1769) (9.932, -15.1698) (9.9306, -15.1628) (9.9293, -15.1559) (9.9279, -15.149) (9.9266, -15.1421) (9.9252, -15.1353) (9.9239, -15.1286) (9.9225, -15.122) (9.9212, -15.1154) (9.9199, -15.1088) (9.9185, -15.1023) (9.9172, -15.0959) (9.9158, -15.0896) (9.9145, -15.0833) (9.9132, -15.077) (9.9118, -15.0709) (9.9105, -15.0647) (9.9092, -15.0587) (9.9079, -15.0527) (9.9065, -15.0468) (9.9052, -15.0409) (9.9039, -15.0352) (9.9026, -15.0294) (9.9013, -15.0238) (9.9, -15.0182) (9.8987, -15.0127) (9.8974, -15.0072) (9.8962, -15.0018) (9.8949, -14.9965) (9.8936, -14.9912) (9.8924, -14.9861) (9.8911, -14.981) (9.8899, -14.9759) (9.8887, -14.9709) (9.8874, -14.966) (9.8862, -14.9612) (9.885, -14.9564) (9.8838, -14.9517) (9.8827, -14.9471) (9.8815, -14.9426) (9.8803, -14.9381) (9.8792, -14.9337) (9.878, -14.9294) (9.8769, -14.9252) (9.8758, -14.921) (9.8747, -14.9169) (9.8736, -14.9129) (9.8725, -14.909) (9.8715, -14.9051) (9.8704, -14.9013) (9.8694, -14.8976) (9.8684, -14.894) (9.8674, -14.8905) (9.8664, -14.887) (9.8654, -14.8837) (9.8645, -14.8804) (9.8635, -14.8772) (9.8626, -14.8741) (9.8617, -14.871) (9.8608, -14.8681) (9.86, -14.8652) (9.8591, -14.8625) (9.8583, -14.8598) (9.8575, -14.8572) (9.8568, -14.8547) (9.856, -14.8523) (9.8553, -14.8499) (9.8546, -14.8477) (9.8539, -14.8456) (9.8533, -14.8435) (9.8527, -14.8416) (9.8521, -14.8398) (9.8515, -14.838) (9.851, -14.8364) (9.8505, -14.8348) (9.85, -14.8334) (9.8495, -14.832) (9.8491, -14.8308) (9.8487, -14.8296) (9.8484, -14.8286) (9.8481, -14.8277) (9.8478, -14.8269) (9.8475, -14.8262) (9.8474, -14.8257) (9.8473, -14.8254) (9.8472, -14.8252) (9.8472, -14.8251) knots -1 -1 -1 -1 -1 -1 -0.99583333 -0.99166667 -0.9875 -0.98333333 -0.97916667 -0.975 -0.97083333 -0.96666667 -0.9625 -0.95833333 -0.95416667 -0.95 -0.94583333 -0.94166667 -0.9375 -0.93333333 -0.92916667 -0.925 -0.92083333 -0.91666667 -0.9125 -0.90833333 -0.90416667 -0.9 -0.89583333 -0.89166667 -0.8875 -0.88333333 -0.87916667 -0.875 -0.87083333 -0.86666667 -0.8625 -0.85833333 -0.85416667 -0.85 -0.84583333 -0.84166667 -0.8375 -0.83333333 -0.82916667 -0.825 -0.82083333 -0.81666667 -0.8125 -0.80833333 -0.80416667 -0.8 -0.79583333 -0.79166667 -0.7875 -0.78333333 -0.77916667 -0.775 -0.77083333 -0.76666667 -0.7625 -0.75833333 -0.75416667 -0.75 -0.74583333 -0.74166667 -0.7375 -0.73333333 -0.72916667 -0.725 -0.72083333 -0.71666667 -0.7125 -0.70833333 -0.70416667 -0.7 -0.69583333 -0.69166667 -0.6875 -0.68333333 -0.67916667 -0.675 -0.67083333 -0.66666667 -0.6625 -0.65833333 -0.65416667 -0.65 -0.64583333 -0.64166667 -0.6375 -0.63333333 -0.62916667 -0.625 -0.62083333 -0.61666667 -0.6125 -0.60833333 -0.60416667 -0.6 -0.59583333 -0.59166667 -0.5875 -0.58333333 -0.57916667 -0.575 -0.57083333 -0.56666667 -0.5625 -0.55833333 -0.55416667 -0.55 -0.54583333 -0.54166667 -0.5375 -0.53333333 -0.52916667 -0.525 -0.52083333 -0.51666667 -0.5125 -0.50833333 -0.50416667 -0.5 -0.49583333 -0.49166667 -0.4875 -0.48333333 -0.47916667 -0.475 -0.47083333 -0.46666667 -0.4625 -0.45833333 -0.45416667 -0.45 -0.44583333 -0.44166667 -0.4375 -0.43333333 -0.42916667 -0.425 -0.42083333 -0.41666667 -0.4125 -0.40833333 -0.40416667 -0.4 -0.39583333 -0.39166667 -0.3875 -0.38333333 -0.37916667 -0.375 -0.37083333 -0.36666667 -0.3625 -0.35833333 -0.35416667 -0.35 -0.34583333 -0.34166667 -0.3375 -0.33333333 -0.32916667 -0.325 -0.32083333 -0.31666667 -0.3125 -0.30833333 -0.30416667 -0.3 -0.29583333 -0.29166667 -0.2875 -0.28333333 -0.27916667 -0.275 -0.27083333 -0.26666667 -0.2625 -0.25833333 -0.25416667 -0.25 -0.24583333 -0.24166667 -0.2375 -0.23333333 -0.22916667 -0.225 -0.22083333 -0.21666667 -0.2125 -0.20833333 -0.20416667 -0.2 -0.19583333 -0.19166667 -0.1875 -0.18333333 -0.17916667 -0.175 -0.17083333 -0.16666667 -0.1625 -0.15833333 -0.15416667 -0.15 -0.14583333 -0.14166667 -0.1375 -0.13333333 -0.12916667 -0.125 -0.12083333 -0.11666667 -0.1125 -0.10833333 -0.10416667 -0.1 -0.09583333 -0.09166667 -0.0875 -0.08333333 -0.07916667 -0.075 -0.07083333 -0.06666667 -0.0625 -0.05833333 -0.05416667 -0.05 -0.04583333 -0.04166667 -0.0375 -0.03333333 -0.02916667 -0.025 -0.02083333 -0.01666667 -0.0125 -0.00833333 -0.00416667 0 0 0 0 0 0
  arc A89 (16.1526, 36.2836) -> (15.1575, 36.9297) centre (0, 12.5) ccw
  spline S88 degree 5 poles (30.9962, 12.9876) (30.9936, 12.9885) (30.9885, 12.9903) (30.9809, 12.993) (30.9707, 12.9966) (30.958, 13.0011) (30.9453, 13.0055) (30.9327, 13.0099) (30.9201, 13.0143) (30.9075, 13.0187) (30.8949, 13.023) (30.8823, 13.0273) (30.8698, 13.0316) (30.8573, 13.0359) (30.8448, 13.0401) (30.8324, 13.0443) (30.82, 13.0485) (30.8076, 13.0526) (30.7952, 13.0568) (30.7828, 13.0609) (30.7705, 13.0649) (30.7582, 13.069) (30.7459, 13.073) (30.7337, 13.077) (30.7215, 13.081) (30.7093, 13.0849) (30.6971, 13.0889) (30.685, 13.0927) (30.6728, 13.0966) (30.6607, 13.1005) (30.6487, 13.1043) (30.6366, 13.1081) (30.6246, 13.1118) (30.6126, 13.1156) (30.6007, 13.1193) (30.5888, 13.123) (30.5769, 13.1267) (30.565, 13.1303) (30.5531, 13.1339) (30.5413, 13.1375) (30.5295, 13.1411) (30.5178, 13.1446) (30.506, 13.1481) (30.4943, 13.1516) (30.4827, 13.1551) (30.471, 13.1585) (30.4594, 13.1619) (30.4478, 13.1653) (30.4362, 13.1687) (30.4247, 13.172) (30.4132, 13.1753) (30.4017, 13.1786) (30.3903, 13.1819) (30.3789, 13.1851) (30.3675, 13.1883) (30.3562, 13.1915) (30.3448, 13.1947) (30.3336, 13.1978) (30.3223, 13.2009) (30.3111, 13.204) (30.2999, 13.2071) (30.2887, 13.2101) (30.2776, 13.2131) (30.2665, 13.2161) (30.2554, 13.2191) (30.2444, 13.222) (30.2334, 13.2249) (30.2224, 13.2278) (30.2114, 13.2307) (30.2005, 13.2335) (30.1897, 13.2364) (30.1788, 13.2391) (30.168, 13.2419) (30.1572, 13.2447) (30.1465, 13.2474) (30.1358, 13.2501) (30.1251, 13.2528) (30.1145, 13.2554) (30.1038, 13.258) (30.0933, 13.2606) (30.0827, 13.2632) (30.0722, 13.2658) (30.0618, 13.2683) (30.0513, 13.2708) (30.0409, 13.2733) (30.0306, 13.2758) (30.0202, 13.2782) (30.0099, 13.2806) (29.9997, 13.283) (29.9895, 13.2854) (29.9793, 13.2877) (29.9691, 13.29) (29.959, 13.2923) (29.949, 13.2946) (29.9389, 13.2969) (29.9289, 13.2991) (29.919, 13.3013) (29.909, 13.3035) (29.8992, 13.3056) (29.8893, 13.3078) (29.8795, 13.3099) (29.8697, 13.312) (29.86, 13.314) (29.8503, 13.3161) (29.8407, 13.3181) (29.8311, 13.3201) (29.8215, 13.3221) (29.812, 13.324) (29.8025, 13.3259) (29.793, 13.3279) (29.7836, 13.3297) (29.7742, 13.3316) (29.7649, 13.3334) (29.7556, 13.3353) (29.7464, 13.3371) (29.7372, 13.3388) (29.728, 13.3406) (29.7189, 13.3423) (29.7098, 13.344) (29.7008, 13.3457) (29.6918, 13.3474) (29.6828, 13.349) (29.6739, 13.3507) (29.6651, 13.3523) (29.6563, 13.3538) (29.6475, 13.3554) (29.6388, 13.3569) (29.6301, 13.3585) (29.6214, 13.36) (29.6128, 13.3614) (29.6043, 13.3629) (29.5958, 13.3643) (29.5873, 13.3657) (29.5789, 13.3671) (29.5706, 13.3685) (29.5623, 13.3698) (29.554, 13.3712) (29.5458, 13.3725) (29.5376, 13.3738) (29.5295, 13.375) (29.5214, 13.3763) (29.5134, 13.3775) (29.5054, 13.3787) (29.4975, 13.3799) (29.4896, 13.3811) (29.4818, 13.3822) (29.474, 13.3834) (29.4663, 13.3845) (29.4586, 13.3856) (29.451, 13.3866) (29.4434, 13.3877) (29.4359, 13.3887) (29.4284, 13.3897) (29.421, 13.3907) (29.4137, 13.3917) (29.4063, 13.3927) (29.3991, 13.3936) (29.3919, 13.3945) (29.3847, 13.3954) (29.3777, 13.3963) (29.3706, 13.3972) (29.3636, 13.398) (29.3567, 13.3989) (29.3498, 13.3997) (29.343, 13.4005) (29.3363, 13.4012) (29.3296, 13.402) (29.323, 13.4027) (29.3164, 13.4035) (29.3099, 13.4042) (29.3034, 13.4049) (29.297, 13.4055) (29.2906, 13.4062) (29.2844, 13.4068) (29.2781, 13.4075) (29.272, 13.4081) (29.2659, 13.4087) (29.2599, 13.4092) (29.2539, 13.4098) (29.248, 13.4103) (29.2421, 13.4109) (29.2363, 13.4114) (29.2306, 13.4119) (29.225, 13.4124) (29.2194, 13.4128) (29.2139, 13.4133) (29.2084, 13.4137) (29.203, 13.4141) (29.1977, 13.4146) (29.1925, 13.415) (29.1873, 13.4153) (29.1822, 13.4157) (29.1771, 13.4161) (29.1722, 13.4164) (29.1673, 13.4167) (29.1624, 13.417) (29.1577, 13.4173) (29.153, 13.4176) (29.1484, 13.4179) (29.1439, 13.4182) (29.1394, 13.4184) (29.135, 13.4186) (29.1307, 13.4189) (29.1265, 13.4191) (29.1223, 13.4193) (29.1183, 13.4195) (29.1143, 13.4197) (29.1103, 13.4198) (29.1065, 13.42) (29.1028, 13.4201) (29.0991, 13.4203) (29.0955, 13.4204) (29.092, 13.4205) (29.0886, 13.4206) (29.0852, 13.4208) (29.082, 13.4208) (29.0788, 13.4209) (29.0758, 13.421) (29.0728, 13.4211) (29.0699, 13.4211) (29.0671, 13.4212) (29.0644, 13.4212) (29.0618, 13.4213) (29.0592, 13.4213) (29.0568, 13.4214) (29.0545, 13.4214) (29.0522, 13.4214) (29.0501, 13.4214) (29.0481, 13.4214) (29.0461, 13.4214) (29.0443, 13.4214) (29.0425, 13.4214) (29.0409, 13.4214) (29.0394, 13.4214) (29.038, 13.4214) (29.0367, 13.4214) (29.0355, 13.4214) (29.0344, 13.4214) (29.0334, 13.4213) (29.0325, 13.4213) (29.0318, 13.4213) (29.0313, 13.4213) (29.0309, 13.4213) (29.0307, 13.4213) (29.0307, 13.4213) knots -1 -1 -1 -1 -1 -1 -0.99583333 -0.99166667 -0.9875 -0.98333333 -0.97916667 -0.975 -0.97083333 -0.96666667 -0.9625 -0.95833333 -0.95416667 -0.95 -0.94583333 -0.94166667 -0.9375 -0.93333333 -0.92916667 -0.925 -0.92083333 -0.91666667 -0.9125 -0.90833333 -0.90416667 -0.9 -0.89583333 -0.89166667 -0.8875 -0.88333333 -0.87916667 -0.875 -0.87083333 -0.86666667 -0.8625 -0.85833333 -0.85416667 -0.85 -0.84583333 -0.84166667 -0.8375 -0.83333333 -0.82916667 -0.825 -0.82083333 -0.81666667 -0.8125 -0.80833333 -0.80416667 -0.8 -0.79583333 -0.79166667 -0.7875 -0.78333333 -0.77916667 -0.775 -0.77083333 -0.76666667 -0.7625 -0.75833333 -0.75416667 -0.75 -0.74583333 -0.74166667 -0.7375 -0.73333333 -0.72916667 -0.725 -0.72083333 -0.71666667 -0.7125 -0.70833333 -0.70416667 -0.7 -0.69583333 -0.69166667 -0.6875 -0.68333333 -0.67916667 -0.675 -0.67083333 -0.66666667 -0.6625 -0.65833333 -0.65416667 -0.65 -0.64583333 -0.64166667 -0.6375 -0.63333333 -0.62916667 -0.625 -0.62083333 -0.61666667 -0.6125 -0.60833333 -0.60416667 -0.6 -0.59583333 -0.59166667 -0.5875 -0.58333333 -0.57916667 -0.575 -0.57083333 -0.56666667 -0.5625 -0.55833333 -0.55416667 -0.55 -0.54583333 -0.54166667 -0.5375 -0.53333333 -0.52916667 -0.525 -0.52083333 -0.51666667 -0.5125 -0.50833333 -0.50416667 -0.5 -0.49583333 -0.49166667 -0.4875 -0.48333333 -0.47916667 -0.475 -0.47083333 -0.46666667 -0.4625 -0.45833333 -0.45416667 -0.45 -0.44583333 -0.44166667 -0.4375 -0.43333333 -0.42916667 -0.425 -0.42083333 -0.41666667 -0.4125 -0.40833333 -0.40416667 -0.4 -0.39583333 -0.39166667 -0.3875 -0.38333333 -0.37916667 -0.375 -0.37083333 -0.36666667 -0.3625 -0.35833333 -0.35416667 -0.35 -0.34583333 -0.34166667 -0.3375 -0.33333333 -0.32916667 -0.325 -0.32083333 -0.31666667 -0.3125 -0.30833333 -0.30416667 -0.3 -0.29583333 -0.29166667 -0.2875 -0.28333333 -0.27916667 -0.275 -0.27083333 -0.26666667 -0.2625 -0.25833333 -0.25416667 -0.25 -0.24583333 -0.24166667 -0.2375 -0.23333333 -0.22916667 -0.225 -0.22083333 -0.21666667 -0.2125 -0.20833333 -0.20416667 -0.2 -0.19583333 -0.19166667 -0.1875 -0.18333333 -0.17916667 -0.175 -0.17083333 -0.16666667 -0.1625 -0.15833333 -0.15416667 -0.15 -0.14583333 -0.14166667 -0.1375 -0.13333333 -0.12916667 -0.125 -0.12083333 -0.11666667 -0.1125 -0.10833333 -0.10416667 -0.1 -0.09583333 -0.09166667 -0.0875 -0.08333333 -0.07916667 -0.075 -0.07083333 -0.06666667 -0.0625 -0.05833333 -0.05416667 -0.05 -0.04583333 -0.04166667 -0.0375 -0.03333333 -0.02916667 -0.025 -0.02083333 -0.01666667 -0.0125 -0.00833333 -0.00416667 0 0 0 0 0 0
  line L171 (0.9213, 41.5298) -> (0.9213, 41.5307)
  arc A90 (2.0967, 41.1734) -> (0.9119, 41.2355) centre (0, 12.5) ccw
  arc A91 (18.5501, 34.4649) -> (17.6281, 35.2115) centre (0, 12.5) ccw
  line L172 (16.3184, 36.5278) -> (16.318, 36.5271)
  line L173 (17.8086, 35.4441) -> (17.8091, 35.4448)
  arc A92 (30.9962, 12.0124) -> (30.9962, 12.9876) centre (0, 12.5) ccw
  line L174 (15.1575, 36.9297) -> (15.3128, 37.1799)
  line L175 (0.9119, 41.2355) -> (0.9213, 41.5298)
  arc A93 (15.9204, 39.0997) -> (15.0758, 39.5873) centre (0, 12.5) ccw
  line L176 (17.6281, 35.2115) -> (17.8086, 35.4441)
  line L177 (16.318, 36.5271) -> (16.1526, 36.2836)
  line L178 (2.1183, 41.4679) -> (2.1182, 41.4671)
  line L179 (2.1182, 41.4671) -> (2.0967, 41.1734)
  arc A94 (3.7249, 43.2754) -> (2.755, 43.3773) centre (0, 12.5) ccw
  arc A95 (0.4876, 43.4962) -> (-0.4876, 43.4962) centre (0, 12.5) ccw